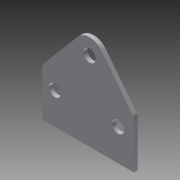
# Autodesk Inventor part: Bracket
Saved by Autodesk Inventor 2014 (Build 180170000, 170)
## iProperties
Created: 2014-01-06
Part Number: Bracket
Material: Aluminum 6061
Document SubType Name: Modeling
Designer: Andrew Toennies
Density: 2.71 g/cm^3
Appearance: Aluminum - Flat
Mass: 4.62013 g
Surface Area: 24.2033 cm^2
Volume: 1.70484 cm^3
Author: Andrew Toennies
Autodesk Inventor part; units mm, degrees
ref_plane "YZ Plane" through (0, 0, 0) normal (1, 0, 0) x (0, 1, 0)
ref_plane "XZ Plane" through (0, 0, 0) normal (0, 1, 0) x (-1, 0, 0)
ref_plane "XY Plane" through (0, 0, 0) normal (0, 0, 1) x (1, 0, 0)
sketch "Sketch1" plane through (0, 0, 0) normal (0, 0, 1) x (1, 0, 0)
  circle A0 centre (0, 0) radius 2.413
  circle A1 centre (25.4, 0) radius 2.413
  line L0 (25.4, 0) -> (0, 0) construction
  line L1 (-5.08, 6.35) -> (31.75, 6.35) construction
  line L2 (31.75, 6.35) -> (31.75, -12.7)
  line L3 (31.75, -12.7) -> (-5.08, -12.7)
  line L4 (-5.08, -12.7) -> (-5.08, 6.35)
  line L5 (-5.08, 6.35) -> (9.1205, 23.1493)
  line L6 (31.75, 6.35) -> (19.0032, 22.9215)
  circle A2 centre (13.97, 19.05) radius 2.4638
  arc A3 (19.0032, 22.9215) -> (9.1205, 23.1493) centre (13.97, 19.05) ccw
  line L7 (-5.08, -12.7) -> (-5.08, 6.35)
  line L8 (-5.08, -12.7) -> (31.75, -12.7)
  line L9 (31.75, -12.7) -> (31.75, 6.35)
  line L10 (31.75, 6.35) -> (19.0032, 22.9215)
  dimension "d1" = 4.826
  dimension "d5" = 12.7
  dimension "d6" = 6.35
  dimension "d7" = 5.08
  dimension "d9" = 6.35
  dimension "d10" = 25.4
  dimension "d14" = 19.05
  dimension "d15" = 12.7
  dimension "d16" = 4.9276
  dimension "d17" = 6.35
  constraints: 22 end point, 4 centre point, 4 equal length, 3 perpendicular, 2 coincident, 2 horizontal, 2 point on circle, 2 tangent, 1 equal radius
  measures "d1" diameter of A1
  measures "d5" distance from line of L3 L0.start
  measures "d6" distance from line of L2 L0.start
  measures "d7" distance from line of L4 point (0, 0)
  measures "d9" distance from line of L1 L0.start
  measures "d10" distance of point (0, 0) L0.start
  measures "d14" distance from line of L4 A2.centre
  measures "d15" distance from line of L1 A2.centre
  measures "d16" diameter of A2
  measures "d17" radius of A3
extrude "Extrusion1" add sketch "Sketch1" along normal blind 1.5875
fillet "Fillet1" radius 3.175 2 edges at (31.75, 6.35, 0.7937) (-5.08, 6.35, 0.7937)
body "Solid1"
